Autodesk Fusion 360 part; units mm, degrees
(part 2 of 15)
  spline S3 degree 5 poles (-5.901, -3.7653) (-5.899, -3.7655) (-5.8948, -3.7657) (-5.8885, -3.7661) (-5.8802, -3.7667) (-5.8698, -3.7673) (-5.8594, -3.7679) (-5.849, -3.7685) (-5.8387, -3.769) (-5.8284, -3.7695) (-5.8181, -3.77) (-5.8079, -3.7705) (-5.7976, -3.7709) (-5.7874, -3.7713) (-5.7772, -3.7717) (-5.7671, -3.772) (-5.757, -3.7724) (-5.7468, -3.7727) (-5.7368, -3.7729) (-5.7267, -3.7732) (-5.7167, -3.7734) (-5.7067, -3.7736) (-5.6967, -3.7738) (-5.6868, -3.7739) (-5.6769, -3.774) (-5.667, -3.7741) (-5.6571, -3.7742) (-5.6473, -3.7742) (-5.6375, -3.7742) (-5.6277, -3.7742) (-5.6179, -3.7741) (-5.6082, -3.7741) (-5.5985, -3.774) (-5.5888, -3.7739) (-5.5792, -3.7737) (-5.5696, -3.7736) (-5.56, -3.7734) (-5.5504, -3.7732) (-5.5409, -3.7729) (-5.5314, -3.7727) (-5.5219, -3.7724) (-5.5125, -3.7721) (-5.5031, -3.7717) (-5.4937, -3.7714) (-5.4843, -3.771) (-5.475, -3.7706) (-5.4657, -3.7702) (-5.4565, -3.7697) (-5.4472, -3.7692) (-5.438, -3.7687) (-5.4289, -3.7682) (-5.4197, -3.7677) (-5.4106, -3.7671) (-5.4015, -3.7665) (-5.3925, -3.7659) (-5.3835, -3.7653) (-5.3745, -3.7646) (-5.3655, -3.764) (-5.3566, -3.7633) (-5.3477, -3.7625) (-5.3389, -3.7618) (-5.33, -3.761) (-5.3212, -3.7603) (-5.3125, -3.7594) (-5.3037, -3.7586) (-5.2951, -3.7578) (-5.2864, -3.7569) (-5.2778, -3.756) (-5.2692, -3.7551) (-5.2606, -3.7542) (-5.2521, -3.7532) (-5.2436, -3.7523) (-5.2351, -3.7513) (-5.2267, -3.7503) (-5.2183, -3.7493) (-5.2099, -3.7482) (-5.2016, -3.7472) (-5.1933, -3.7461) (-5.1851, -3.745) (-5.1768, -3.7439) (-5.1687, -3.7427) (-5.1605, -3.7416) (-5.1524, -3.7404) (-5.1443, -3.7392) (-5.1363, -3.738) (-5.1283, -3.7368) (-5.1203, -3.7355) (-5.1123, -3.7343) (-5.1044, -3.733) (-5.0966, -3.7317) (-5.0887, -3.7304) (-5.081, -3.7291) (-5.0732, -3.7277) (-5.0655, -3.7264) (-5.0578, -3.725) (-5.0502, -3.7236) (-5.0426, -3.7222) (-5.035, -3.7208) (-5.0275, -3.7194) (-5.02, -3.7179) (-5.0125, -3.7165) (-5.0051, -3.715) (-4.9977, -3.7135) (-4.9904, -3.712) (-4.9831, -3.7105) (-4.9758, -3.7089) (-4.9686, -3.7074) (-4.9614, -3.7058) (-4.9543, -3.7043) (-4.9472, -3.7027) (-4.9401, -3.7011) (-4.9331, -3.6995) (-4.9261, -3.6978) (-4.9191, -3.6962) (-4.9122, -3.6946) (-4.9054, -3.6929) (-4.8986, -3.6912) (-4.8918, -3.6896) (-4.885, -3.6879) (-4.8783, -3.6862) (-4.8717, -3.6845) (-4.8651, -3.6827) (-4.8585, -3.681) (-4.8519, -3.6793) (-4.8454, -3.6775) (-4.839, -3.6758) (-4.8326, -3.674) (-4.8262, -3.6722) (-4.8199, -3.6705) (-4.8136, -3.6687) (-4.8074, -3.6669) (-4.8012, -3.6651) (-4.795, -3.6632) (-4.7889, -3.6614) (-4.7829, -3.6596) (-4.7768, -3.6578) (-4.7709, -3.6559) (-4.7649, -3.6541) (-4.759, -3.6522) (-4.7532, -3.6504) (-4.7474, -3.6485) (-4.7416, -3.6466) (-4.7359, -3.6448) (-4.7303, -3.6429) (-4.7246, -3.641) (-4.7191, -3.6391) (-4.7135, -3.6373) (-4.708, -3.6354) (-4.7026, -3.6335) (-4.6972, -3.6316) (-4.6919, -3.6297) (-4.6866, -3.6278) (-4.6813, -3.6259) (-4.6761, -3.624) (-4.6709, -3.6221) (-4.6658, -3.6202) (-4.6608, -3.6183) (-4.6557, -3.6164) (-4.6508, -3.6145) (-4.6458, -3.6126) (-4.641, -3.6107) (-4.6361, -3.6088) (-4.6314, -3.6069) (-4.6266, -3.605) (-4.6219, -3.6031) (-4.6173, -3.6012) (-4.6127, -3.5993) (-4.6082, -3.5974) (-4.6037, -3.5955) (-4.5993, -3.5937) (-4.5949, -3.5918) (-4.5905, -3.5899) (-4.5863, -3.5881) (-4.582, -3.5862) (-4.5778, -3.5843) (-4.5737, -3.5825) (-4.5696, -3.5807) (-4.5656, -3.5788) (-4.5616, -3.577) (-4.5577, -3.5752) (-4.5538, -3.5734) (-4.5499, -3.5716) (-4.5462, -3.5698) (-4.5424, -3.568) (-4.5388, -3.5663) (-4.5351, -3.5645) (-4.5316, -3.5628) (-4.5281, -3.561) (-4.5246, -3.5593) (-4.5212, -3.5576) (-4.5178, -3.5559) (-4.5145, -3.5542) (-4.5113, -3.5525) (-4.5081, -3.5509) (-4.5049, -3.5492) (-4.5018, -3.5476) (-4.4988, -3.546) (-4.4958, -3.5444) (-4.4929, -3.5428) (-4.49, -3.5413) (-4.4872, -3.5397) (-4.4845, -3.5382) (-4.4818, -3.5367) (-4.4791, -3.5352) (-4.4765, -3.5338) (-4.474, -3.5323) (-4.4715, -3.5309) (-4.4691, -3.5295) (-4.4667, -3.5281) (-4.4644, -3.5267) (-4.4622, -3.5254) (-4.46, -3.5241) (-4.4579, -3.5228) (-4.4558, -3.5215) (-4.4538, -3.5203) (-4.4518, -3.5191) (-4.4499, -3.5179) (-4.4481, -3.5168) (-4.4463, -3.5156) (-4.4446, -3.5145) (-4.4429, -3.5135) (-4.4413, -3.5124) (-4.4398, -3.5114) (-4.4383, -3.5104) (-4.4369, -3.5095) (-4.4355, -3.5086) (-4.4342, -3.5077) (-4.433, -3.5069) (-4.4318, -3.5061) (-4.4307, -3.5053) (-4.4296, -3.5046) (-4.4286, -3.5039) (-4.4277, -3.5032) (-4.4268, -3.5026) (-4.426, -3.502) (-4.4253, -3.5015) (-4.4246, -3.501) (-4.424, -3.5005) (-4.4234, -3.5001) (-4.423, -3.4998) (-4.4225, -3.4994) (-4.4222, -3.4992) (-4.4221, -3.4991) (-4.422, -3.499) (-4.4219, -3.499) knots -1 -1 -1 -1 -1 -1 -0.99583333 -0.99166667 -0.9875 -0.98333333 -0.97916667 -0.975 -0.97083333 -0.96666667 -0.9625 -0.95833333 -0.95416667 -0.95 -0.94583333 -0.94166667 -0.9375 -0.93333333 -0.92916667 -0.925 -0.92083333 -0.91666667 -0.9125 -0.90833333 -0.90416667 -0.9 -0.89583333 -0.89166667 -0.8875 -0.88333333 -0.87916667 -0.875 -0.87083333 -0.86666667 -0.8625 -0.85833333 -0.85416667 -0.85 -0.84583333 -0.84166667 -0.8375 -0.83333333 -0.82916667 -0.825 -0.82083333 -0.81666667 -0.8125 -0.80833333 -0.80416667 -0.8 -0.79583333 -0.79166667 -0.7875 -0.78333333 -0.77916667 -0.775 -0.77083333 -0.76666667 -0.7625 -0.75833333 -0.75416667 -0.75 -0.74583333 -0.74166667 -0.7375 -0.73333333 -0.72916667 -0.725 -0.72083333 -0.71666667 -0.7125 -0.70833333 -0.70416667 -0.7 -0.69583333 -0.69166667 -0.6875 -0.68333333 -0.67916667 -0.675 -0.67083333 -0.66666667 -0.6625 -0.65833333 -0.65416667 -0.65 -0.64583333 -0.64166667 -0.6375 -0.63333333 -0.62916667 -0.625 -0.62083333 -0.61666667 -0.6125 -0.60833333 -0.60416667 -0.6 -0.59583333 -0.59166667 -0.5875 -0.58333333 -0.57916667 -0.575 -0.57083333 -0.56666667 -0.5625 -0.55833333 -0.55416667 -0.55 -0.54583333 -0.54166667 -0.5375 -0.53333333 -0.52916667 -0.525 -0.52083333 -0.51666667 -0.5125 -0.50833333 -0.50416667 -0.5 -0.49583333 -0.49166667 -0.4875 -0.48333333 -0.47916667 -0.475 -0.47083333 -0.46666667 -0.4625 -0.45833333 -0.45416667 -0.45 -0.44583333 -0.44166667 -0.4375 -0.43333333 -0.42916667 -0.425 -0.42083333 -0.41666667 -0.4125 -0.40833333 -0.40416667 -0.4 -0.39583333 -0.39166667 -0.3875 -0.38333333 -0.37916667 -0.375 -0.37083333 -0.36666667 -0.3625 -0.35833333 -0.35416667 -0.35 -0.34583333 -0.34166667 -0.3375 -0.33333333 -0.32916667 -0.325 -0.32083333 -0.31666667 -0.3125 -0.30833333 -0.30416667 -0.3 -0.29583333 -0.29166667 -0.2875 -0.28333333 -0.27916667 -0.275 -0.27083333 -0.26666667 -0.2625 -0.25833333 -0.25416667 -0.25 -0.24583333 -0.24166667 -0.2375 -0.23333333 -0.22916667 -0.225 -0.22083333 -0.21666667 -0.2125 -0.20833333 -0.20416667 -0.2 -0.19583333 -0.19166667 -0.1875 -0.18333333 -0.17916667 -0.175 -0.17083333 -0.16666667 -0.1625 -0.15833333 -0.15416667 -0.15 -0.14583333 -0.14166667 -0.1375 -0.13333333 -0.12916667 -0.125 -0.12083333 -0.11666667 -0.1125 -0.10833333 -0.10416667 -0.1 -0.09583333 -0.09166667 -0.0875 -0.08333333 -0.07916667 -0.075 -0.07083333 -0.06666667 -0.0625 -0.05833333 -0.05416667 -0.05 -0.04583333 -0.04166667 -0.0375 -0.03333333 -0.02916667 -0.025 -0.02083333 -0.01666667 -0.0125 -0.00833333 -0.00416667 0 0 0 0 0 0
  line L6 (-4.4219, -3.499) -> (-4.4214, -3.4986)
  line L7 (-4.4214, -3.4986) -> (-3.7249, -2.9475)
  arc A4 (-3.7249, -2.9475) -> (-2.9475, -3.7249) centre (0, 0) ccw
  line L8 (-2.9475, -3.7249) -> (-3.4986, -4.4214)
  line L9 (-3.4986, -4.4214) -> (-3.499, -4.4219)
  spline S4 degree 5 poles (-3.499, -4.4219) (-3.499, -4.422) (-3.4991, -4.4221) (-3.4992, -4.4222) (-3.4994, -4.4225) (-3.4998, -4.423) (-3.5001, -4.4234) (-3.5005, -4.424) (-3.501, -4.4246) (-3.5015, -4.4253) (-3.502, -4.426) (-3.5026, -4.4268) (-3.5032, -4.4277) (-3.5039, -4.4286) (-3.5046, -4.4296) (-3.5053, -4.4307) (-3.5061, -4.4318) (-3.5069, -4.433) (-3.5077, -4.4342) (-3.5086, -4.4355) (-3.5095, -4.4369) (-3.5104, -4.4383) (-3.5114, -4.4398) (-3.5124, -4.4413) (-3.5135, -4.4429) (-3.5145, -4.4446) (-3.5156, -4.4463) (-3.5168, -4.4481) (-3.5179, -4.4499) (-3.5191, -4.4518) (-3.5203, -4.4538) (-3.5215, -4.4558) (-3.5228, -4.4579) (-3.5241, -4.46) (-3.5254, -4.4622) (-3.5267, -4.4644) (-3.5281, -4.4667) (-3.5295, -4.4691) (-3.5309, -4.4715) (-3.5323, -4.474) (-3.5338, -4.4765) (-3.5352, -4.4791) (-3.5367, -4.4818) (-3.5382, -4.4845) (-3.5397, -4.4872) (-3.5413, -4.49) (-3.5428, -4.4929) (-3.5444, -4.4958) (-3.546, -4.4988) (-3.5476, -4.5018) (-3.5492, -4.5049) (-3.5509, -4.5081) (-3.5525, -4.5113) (-3.5542, -4.5145) (-3.5559, -4.5178) (-3.5576, -4.5212) (-3.5593, -4.5246) (-3.561, -4.5281) (-3.5628, -4.5316) (-3.5645, -4.5351) (-3.5663, -4.5388) (-3.568, -4.5424) (-3.5698, -4.5462) (-3.5716, -4.5499) (-3.5734, -4.5538) (-3.5752, -4.5577) (-3.577, -4.5616) (-3.5788, -4.5656) (-3.5807, -4.5696) (-3.5825, -4.5737) (-3.5843, -4.5778) (-3.5862, -4.582) (-3.5881, -4.5863) (-3.5899, -4.5905) (-3.5918, -4.5949) (-3.5937, -4.5993) (-3.5955, -4.6037) (-3.5974, -4.6082) (-3.5993, -4.6127) (-3.6012, -4.6173) (-3.6031, -4.6219) (-3.605, -4.6266) (-3.6069, -4.6314) (-3.6088, -4.6361) (-3.6107, -4.641) (-3.6126, -4.6458) (-3.6145, -4.6508) (-3.6164, -4.6557) (-3.6183, -4.6608) (-3.6202, -4.6658) (-3.6221, -4.6709) (-3.624, -4.6761) (-3.6259, -4.6813) (-3.6278, -4.6866) (-3.6297, -4.6919) (-3.6316, -4.6972) (-3.6335, -4.7026) (-3.6354, -4.708) (-3.6373, -4.7135) (-3.6391, -4.7191) (-3.641, -4.7246) (-3.6429, -4.7303) (-3.6448, -4.7359) (-3.6466, -4.7416) (-3.6485, -4.7474) (-3.6504, -4.7532) (-3.6522, -4.759) (-3.6541, -4.7649) (-3.6559, -4.7709) (-3.6578, -4.7768) (-3.6596, -4.7829) (-3.6614, -4.7889) (-3.6632, -4.795) (-3.6651, -4.8012) (-3.6669, -4.8074) (-3.6687, -4.8136) (-3.6705, -4.8199) (-3.6722, -4.8262) (-3.674, -4.8326) (-3.6758, -4.839) (-3.6775, -4.8454) (-3.6793, -4.8519) (-3.681, -4.8585) (-3.6827, -4.8651) (-3.6845, -4.8717) (-3.6862, -4.8783) (-3.6879, -4.885) (-3.6896, -4.8918) (-3.6912, -4.8986) (-3.6929, -4.9054) (-3.6946, -4.9122) (-3.6962, -4.9191) (-3.6978, -4.9261) (-3.6995, -4.9331) (-3.7011, -4.9401) (-3.7027, -4.9472) (-3.7043, -4.9543) (-3.7058, -4.9614) (-3.7074, -4.9686) (-3.7089, -4.9758) (-3.7105, -4.9831) (-3.712, -4.9904) (-3.7135, -4.9977) (-3.715, -5.0051) (-3.7165, -5.0125) (-3.7179, -5.02) (-3.7194, -5.0275) (-3.7208, -5.035) (-3.7222, -5.0426) (-3.7236, -5.0502) (-3.725, -5.0578) (-3.7264, -5.0655) (-3.7277, -5.0732) (-3.7291, -5.081) (-3.7304, -5.0887) (-3.7317, -5.0966) (-3.733, -5.1044) (-3.7343, -5.1123) (-3.7355, -5.1203) (-3.7368, -5.1283) (-3.738, -5.1363) (-3.7392, -5.1443) (-3.7404, -5.1524) (-3.7416, -5.1605) (-3.7427, -5.1687) (-3.7439, -5.1768) (-3.745, -5.1851) (-3.7461, -5.1933) (-3.7472, -5.2016) (-3.7482, -5.2099) (-3.7493, -5.2183) (-3.7503, -5.2267) (-3.7513, -5.2351) (-3.7523, -5.2436) (-3.7532, -5.2521) (-3.7542, -5.2606) (-3.7551, -5.2692) (-3.756, -5.2778) (-3.7569, -5.2864) (-3.7578, -5.2951) (-3.7586, -5.3037) (-3.7594, -5.3125) (-3.7603, -5.3212) (-3.761, -5.33) (-3.7618, -5.3389) (-3.7625, -5.3477) (-3.7633, -5.3566) (-3.764, -5.3655) (-3.7646, -5.3745) (-3.7653, -5.3835) (-3.7659, -5.3925) (-3.7665, -5.4015) (-3.7671, -5.4106) (-3.7677, -5.4197) (-3.7682, -5.4289) (-3.7687, -5.438) (-3.7692, -5.4472) (-3.7697, -5.4565) (-3.7702, -5.4657) (-3.7706, -5.475) (-3.771, -5.4843) (-3.7714, -5.4937) (-3.7717, -5.5031) (-3.7721, -5.5125) (-3.7724, -5.5219) (-3.7727, -5.5314) (-3.7729, -5.5409) (-3.7732, -5.5504) (-3.7734, -5.56) (-3.7736, -5.5696) (-3.7737, -5.5792) (-3.7739, -5.5888) (-3.774, -5.5985) (-3.7741, -5.6082) (-3.7741, -5.6179) (-3.7742, -5.6277) (-3.7742, -5.6375) (-3.7742, -5.6473) (-3.7742, -5.6571) (-3.7741, -5.667) (-3.774, -5.6769) (-3.7739, -5.6868) (-3.7738, -5.6967) (-3.7736, -5.7067) (-3.7734, -5.7167) (-3.7732, -5.7267) (-3.7729, -5.7368) (-3.7727, -5.7468) (-3.7724, -5.757) (-3.772, -5.7671) (-3.7717, -5.7772) (-3.7713, -5.7874) (-3.7709, -5.7976) (-3.7705, -5.8079) (-3.77, -5.8181) (-3.7695, -5.8284) (-3.769, -5.8387) (-3.7685, -5.849) (-3.7679, -5.8594) (-3.7673, -5.8698) (-3.7667, -5.8802) (-3.7661, -5.8885) (-3.7657, -5.8948) (-3.7655, -5.899) (-3.7653, -5.901) knots 0 0 0 0 0 0 0.00416667 0.00833333 0.0125 0.01666667 0.02083333 0.025 0.02916667 0.03333333 0.0375 0.04166667 0.04583333 0.05 0.05416667 0.05833333 0.0625 0.06666667 0.07083333 0.075 0.07916667 0.08333333 0.0875 0.09166667 0.09583333 0.1 0.10416667 0.10833333 0.1125 0.11666667 0.12083333 0.125 0.12916667 0.13333333 0.1375 0.14166667 0.14583333 0.15 0.15416667 0.15833333 0.1625 0.16666667 0.17083333 0.175 0.17916667 0.18333333 0.1875 0.19166667 0.19583333 0.2 0.20416667 0.20833333 0.2125 0.21666667 0.22083333 0.225 0.22916667 0.23333333 0.2375 0.24166667 0.24583333 0.25 0.25416667 0.25833333 0.2625 0.26666667 0.27083333 0.275 0.27916667 0.28333333 0.2875 0.29166667 0.29583333 0.3 0.30416667 0.30833333 0.3125 0.31666667 0.32083333 0.325 0.32916667 0.33333333 0.3375 0.34166667 0.34583333 0.35 0.35416667 0.35833333 0.3625 0.36666667 0.37083333 0.375 0.37916667 0.38333333 0.3875 0.39166667 0.39583333 0.4 0.40416667 0.40833333 0.4125 0.41666667 0.42083333 0.425 0.42916667 0.43333333 0.4375 0.44166667 0.44583333 0.45 0.45416667 0.45833333 0.4625 0.46666667 0.47083333 0.475 0.47916667 0.48333333 0.4875 0.49166667 0.49583333 0.5 0.50416667 0.50833333 0.5125 0.51666667 0.52083333 0.525 0.52916667 0.53333333 0.5375 0.54166667 0.54583333 0.55 0.55416667 0.55833333 0.5625 0.56666667 0.57083333 0.575 0.57916667 0.58333333 0.5875 0.59166667 0.59583333 0.6 0.60416667 0.60833333 0.6125 0.61666667 0.62083333 0.625 0.62916667 0.63333333 0.6375 0.64166667 0.64583333 0.65 0.65416667 0.65833333 0.6625 0.66666667 0.67083333 0.675 0.67916667 0.68333333 0.6875 0.69166667 0.69583333 0.7 0.70416667 0.70833333 0.7125 0.71666667 0.72083333 0.725 0.72916667 0.73333333 0.7375 0.74166667 0.74583333 0.75 0.75416667 0.75833333 0.7625 0.76666667 0.77083333 0.775 0.77916667 0.78333333 0.7875 0.79166667 0.79583333 0.8 0.80416667 0.80833333 0.8125 0.81666667 0.82083333 0.825 0.82916667 0.83333333 0.8375 0.84166667 0.84583333 0.85 0.85416667 0.85833333 0.8625 0.86666667 0.87083333 0.875 0.87916667 0.88333333 0.8875 0.89166667 0.89583333 0.9 0.90416667 0.90833333 0.9125 0.91666667 0.92083333 0.925 0.92916667 0.93333333 0.9375 0.94166667 0.94583333 0.95 0.95416667 0.95833333 0.9625 0.96666667 0.97083333 0.975 0.97916667 0.98333333 0.9875 0.99166667 0.99583333 1 1 1 1 1 1
  arc A5 (-3.7653, -5.901) -> (-3.2278, -6.2114) centre (0, 0) ccw
  spline S5 degree 5 poles (-3.2278, -6.2114) (-3.2259, -6.2105) (-3.2221, -6.2086) (-3.2165, -6.2058) (-3.209, -6.2021) (-3.1997, -6.1975) (-3.1904, -6.1928) (-3.1812, -6.1881) (-3.172, -6.1834) (-3.1628, -6.1787) (-3.1536, -6.174) (-3.1445, -6.1692) (-3.1354, -6.1645) (-3.1264, -6.1598) (-3.1174, -6.155) (-3.1084, -6.1502) (-3.0995, -6.1454) (-3.0906, -6.1406) (-3.0817, -6.1358) (-3.0729, -6.131) (-3.0641, -6.1262) (-3.0554, -6.1214) (-3.0466, -6.1165) (-3.038, -6.1117) (-3.0293, -6.1068) (-3.0207, -6.1019) (-3.0121, -6.0971) (-3.0036, -6.0922) (-2.9951, -6.0873) (-2.9866, -6.0824) (-2.9782, -6.0775) (-2.9698, -6.0726) (-2.9614, -6.0676) (-2.9531, -6.0627) (-2.9448, -6.0577) (-2.9366, -6.0528) (-2.9284, -6.0478) (-2.9202, -6.0429) (-2.9121, -6.0379) (-2.904, -6.0329) (-2.8959, -6.0279) (-2.8879, -6.023) (-2.8799, -6.018) (-2.872, -6.013) (-2.8641, -6.008) (-2.8562, -6.0029) (-2.8484, -5.9979) (-2.8406, -5.9929) (-2.8328, -5.9879) (-2.8251, -5.9828) (-2.8174, -5.9778) (-2.8098, -5.9728) (-2.8022, -5.9677) (-2.7946, -5.9627) (-2.7871, -5.9576) (-2.7796, -5.9526) (-2.7721, -5.9475) (-2.7647, -5.9424) (-2.7573, -5.9374) (-2.75, -5.9323) (-2.7427, -5.9272) (-2.7354, -5.9222) (-2.7282, -5.9171) (-2.721, -5.912) (-2.7139, -5.9069) (-2.7068, -5.9019) (-2.6997, -5.8968) (-2.6927, -5.8917) (-2.6857, -5.8866) (-2.6787, -5.8815) (-2.6718, -5.8764) (-2.6649, -5.8714) (-2.6581, -5.8663) (-2.6513, -5.8612) (-2.6445, -5.8561) (-2.6378, -5.851) (-2.6311, -5.8459) (-2.6245, -5.8409) (-2.6179, -5.8358) (-2.6113, -5.8307) (-2.6048, -5.8256) (-2.5983, -5.8205) (-2.5919, -5.8155) (-2.5855, -5.8104) (-2.5791, -5.8053) (-2.5728, -5.8003) (-2.5665, -5.7952) (-2.5603, -5.7902) (-2.5541, -5.7851) (-2.5479, -5.78) (-2.5418, -5.775) (-2.5357, -5.77) (-2.5297, -5.7649) (-2.5236, -5.7599) (-2.5177, -5.7549) (-2.5118, -5.7498) (-2.5059, -5.7448) (-2.5, -5.7398) (-2.4942, -5.7348) (-2.4885, -5.7298) (-2.4827, -5.7248) (-2.4771, -5.7198) (-2.4714, -5.7148) (-2.4658, -5.7099) (-2.4602, -5.7049) (-2.4547, -5.6999) (-2.4492, -5.695) (-2.4438, -5.69) (-2.4384, -5.6851) (-2.433, -5.6802) (-2.4277, -5.6753) (-2.4224, -5.6704) (-2.4172, -5.6655) (-2.412, -5.6606) (-2.4068, -5.6557) (-2.4017, -5.6508) (-2.3967, -5.646) (-2.3916, -5.6411) (-2.3866, -5.6363) (-2.3817, -5.6315) (-2.3768, -5.6267) (-2.3719, -5.6219) (-2.3671, -5.6171) (-2.3623, -5.6123) (-2.3575, -5.6076) (-2.3528, -5.6028) (-2.3481, -5.5981) (-2.3435, -5.5934) (-2.3389, -5.5887) (-2.3344, -5.584) (-2.3299, -5.5793) (-2.3254, -5.5746) (-2.321, -5.57) (-2.3166, -5.5653) (-2.3123, -5.5607) (-2.308, -5.5561) (-2.3037, -5.5516) (-2.2995, -5.547) (-2.2953, -5.5424) (-2.2912, -5.5379) (-2.2871, -5.5334) (-2.283, -5.5289) (-2.279, -5.5244) (-2.2751, -5.52) (-2.2711, -5.5155) (-2.2673, -5.5111) (-2.2634, -5.5067) (-2.2596, -5.5023) (-2.2558, -5.498) (-2.2521, -5.4936) (-2.2484, -5.4893) (-2.2448, -5.485) (-2.2412, -5.4808) (-2.2376, -5.4765) (-2.2341, -5.4723) (-2.2306, -5.4681) (-2.2272, -5.4639) (-2.2238, -5.4597) (-2.2204, -5.4556) (-2.2171, -5.4515) (-2.2139, -5.4474) (-2.2106, -5.4434) (-2.2074, -5.4393) (-2.2043, -5.4353) (-2.2012, -5.4313) (-2.1981, -5.4274) (-2.1951, -5.4234) (-2.1921, -5.4195) (-2.1892, -5.4157) (-2.1863, -5.4118) (-2.1834, -5.408) (-2.1806, -5.4042) (-2.1778, -5.4005) (-2.175, -5.3967) (-2.1723, -5.393) (-2.1697, -5.3894) (-2.1671, -5.3858) (-2.1645, -5.3821) (-2.1619, -5.3786) (-2.1594, -5.375) (-2.157, -5.3715) (-2.1546, -5.3681) (-2.1522, -5.3646) (-2.1498, -5.3612) (-2.1475, -5.3579) (-2.1453, -5.3545) (-2.1431, -5.3512) (-2.1409, -5.348) (-2.1388, -5.3447) (-2.1367, -5.3416) (-2.1346, -5.3384) (-2.1326, -5.3353) (-2.1306, -5.3322) (-2.1287, -5.3292) (-2.1268, -5.3262) (-2.1249, -5.3233) (-2.1231, -5.3203) (-2.1213, -5.3175) (-2.1196, -5.3146) (-2.1179, -5.3119) (-2.1162, -5.3091) (-2.1146, -5.3064) (-2.113, -5.3038) (-2.1114, -5.3012) (-2.1099, -5.2986) (-2.1084, -5.2961) (-2.107, -5.2936) (-2.1056, -5.2912) (-2.1043, -5.2888) (-2.1029, -5.2865) (-2.1017, -5.2842) (-2.1004, -5.2819) (-2.0992, -5.2798) (-2.0981, -5.2776) (-2.0969, -5.2756) (-2.0958, -5.2735) (-2.0948, -5.2716) (-2.0938, -5.2696) (-2.0928, -5.2678) (-2.0918, -5.266) (-2.0909, -5.2642) (-2.0901, -5.2625) (-2.0892, -5.2609) (-2.0884, -5.2593) (-2.0877, -5.2577) (-2.087, -5.2563) (-2.0863, -5.2549) (-2.0856, -5.2535) (-2.085, -5.2522) (-2.0844, -5.251) (-2.0839, -5.2498) (-2.0834, -5.2487) (-2.0829, -5.2477) (-2.0824, -5.2467) (-2.082, -5.2458) (-2.0817, -5.245) (-2.0813, -5.2442) (-2.081, -5.2435) (-2.0807, -5.2429) (-2.0805, -5.2424) (-2.0803, -5.2419) (-2.0802, -5.2415) (-2.0801, -5.2413) (-2.08, -5.2412) (-2.08, -5.2411) knots -1 -1 -1 -1 -1 -1 -0.99583333 -0.99166667 -0.9875 -0.98333333 -0.97916667 -0.975 -0.97083333 -0.96666667 -0.9625 -0.95833333 -0.95416667 -0.95 -0.94583333 -0.94166667 -0.9375 -0.93333333 -0.92916667 -0.925 -0.92083333 -0.91666667 -0.9125 -0.90833333 -0.90416667 -0.9 -0.89583333 -0.89166667 -0.8875 -0.88333333 -0.87916667 -0.875 -0.87083333 -0.86666667 -0.8625 -0.85833333 -0.85416667 -0.85 -0.84583333 -0.84166667 -0.8375 -0.83333333 -0.82916667 -0.825 -0.82083333 -0.81666667 -0.8125 -0.80833333 -0.80416667 -0.8 -0.79583333 -0.79166667 -0.7875 -0.78333333 -0.77916667 -0.775 -0.77083333 -0.76666667 -0.7625 -0.75833333 -0.75416667 -0.75 -0.74583333 -0.74166667 -0.7375 -0.73333333 -0.72916667 -0.725 -0.72083333 -0.71666667 -0.7125 -0.70833333 -0.70416667 -0.7 -0.69583333 -0.69166667 -0.6875 -0.68333333 -0.67916667 -0.675 -0.67083333 -0.66666667 -0.6625 -0.65833333 -0.65416667 -0.65 -0.64583333 -0.64166667 -0.6375 -0.63333333 -0.62916667 -0.625 -0.62083333 -0.61666667 -0.6125 -0.60833333 -0.60416667 -0.6 -0.59583333 -0.59166667 -0.5875 -0.58333333 -0.57916667 -0.575 -0.57083333 -0.56666667 -0.5625 -0.55833333 -0.55416667 -0.55 -0.54583333 -0.54166667 -0.5375 -0.53333333 -0.52916667 -0.525 -0.52083333 -0.51666667 -0.5125 -0.50833333 -0.50416667 -0.5 -0.49583333 -0.49166667 -0.4875 -0.48333333 -0.47916667 -0.475 -0.47083333 -0.46666667 -0.4625 -0.45833333 -0.45416667 -0.45 -0.44583333 -0.44166667 -0.4375 -0.43333333 -0.42916667 -0.425 -0.42083333 -0.41666667 -0.4125 -0.40833333 -0.40416667 -0.4 -0.39583333 -0.39166667 -0.3875 -0.38333333 -0.37916667 -0.375 -0.37083333 -0.36666667 -0.3625 -0.35833333 -0.35416667 -0.35 -0.34583333 -0.34166667 -0.3375 -0.33333333 -0.32916667 -0.325 -0.32083333 -0.31666667 -0.3125 -0.30833333 -0.30416667 -0.3 -0.29583333 -0.29166667 -0.2875 -0.28333333 -0.27916667 -0.275 -0.27083333 -0.26666667 -0.2625 -0.25833333 -0.25416667 -0.25 -0.24583333 -0.24166667 -0.2375 -0.23333333 -0.22916667 -0.225 -0.22083333 -0.21666667 -0.2125 -0.20833333 -0.20416667 -0.2 -0.19583333 -0.19166667 -0.1875 -0.18333333 -0.17916667 -0.175 -0.17083333 -0.16666667 -0.1625 -0.15833333 -0.15416667 -0.15 -0.14583333 -0.14166667 -0.1375 -0.13333333 -0.12916667 -0.125 -0.12083333 -0.11666667 -0.1125 -0.10833333 -0.10416667 -0.1 -0.09583333 -0.09166667 -0.0875 -0.08333333 -0.07916667 -0.075 -0.07083333 -0.06666667 -0.0625 -0.05833333 -0.05416667 -0.05 -0.04583333 -0.04166667 -0.0375 -0.03333333 -0.02916667 -0.025 -0.02083333 -0.01666667 -0.0125 -0.00833333 -0.00416667 0 0 0 0 0 0
  line L10 (-2.08, -5.2411) -> (-2.0798, -5.2406)
  line L11 (-2.0798, -5.2406) -> (-1.7521, -4.415)
  arc A6 (-1.7521, -4.415) -> (-0.6901, -4.6996) centre (0, 0) ccw
  line L12 (-0.6901, -4.6996) -> (-0.8192, -5.5783)
  line L13 (-0.8192, -5.5783) -> (-0.8192, -5.579)
  spline S6 degree 5 poles (-0.8192, -5.579) (-0.8193, -5.579) (-0.8193, -5.5792) (-0.8193, -5.5794) (-0.8193, -5.5797) (-0.8194, -5.5803) (-0.8195, -5.5809) (-0.8196, -5.5815) (-0.8196, -5.5823) (-0.8197, -5.5831) (-0.8198, -5.584) (-0.8199, -5.585) (-0.82, -5.5861) (-0.8201, -5.5872) (-0.8202, -5.5884) (-0.8203, -5.5897) (-0.8204, -5.5911) (-0.8206, -5.5925) (-0.8207, -5.594) (-0.8208, -5.5955) (-0.8209, -5.5972) (-0.821, -5.5989) (-0.8211, -5.6007) (-0.8212, -5.6025) (-0.8213, -5.6044) (-0.8214, -5.6064) (-0.8215, -5.6084) (-0.8216, -5.6105) (-0.8216, -5.6127) (-0.8217, -5.6149) (-0.8218, -5.6172) (-0.8218, -5.6196) (-0.8219, -5.622) (-0.822, -5.6245) (-0.822, -5.6271) (-0.822, -5.6297) (-0.822, -5.6324) (-0.8221, -5.6351) (-0.8221, -5.6379) (-0.8221, -5.6408) (-0.8221, -5.6437) (-0.822, -5.6466) (-0.822, -5.6497) (-0.8219, -5.6528) (-0.8219, -5.6559) (-0.8218, -5.6591) (-0.8217, -5.6624) (-0.8216, -5.6657) (-0.8215, -5.6691) (-0.8214, -5.6725) (-0.8213, -5.676) (-0.8211, -5.6796) (-0.821, -5.6831) (-0.8208, -5.6868) (-0.8206, -5.6905) (-0.8204, -5.6943) (-0.8202, -5.6981) (-0.8199, -5.7019) (-0.8197, -5.7058) (-0.8194, -5.7098) (-0.8191, -5.7138) (-0.8188, -5.7179) (-0.8185, -5.722) (-0.8181, -5.7262) (-0.8178, -5.7304) (-0.8174, -5.7346) (-0.817, -5.739) (-0.8166, -5.7433) (-0.8161, -5.7477) (-0.8157, -5.7522) (-0.8152, -5.7567) (-0.8147, -5.7612) (-0.8142, -5.7658) (-0.8137, -5.7705) (-0.8131, -5.7752) (-0.8126, -5.7799) (-0.812, -5.7847) (-0.8114, -5.7895) (-0.8107, -5.7944) (-0.8101, -5.7993) (-0.8094, -5.8043) (-0.8087, -5.8093) (-0.808, -5.8143) (-0.8072, -5.8194) (-0.8064, -5.8245) (-0.8057, -5.8297) (-0.8048, -5.8349) (-0.804, -5.8402) (-0.8031, -5.8455) (-0.8023, -5.8508) (-0.8013, -5.8562) (-0.8004, -5.8616) (-0.7995, -5.8671) (-0.7985, -5.8726) (-0.7975, -5.8781) (-0.7964, -5.8837) (-0.7954, -5.8893) (-0.7943, -5.895) (-0.7932, -5.9007) (-0.7921, -5.9064) (-0.7909, -5.9122) (-0.7897, -5.918) (-0.7885, -5.9238) (-0.7873, -5.9297) (-0.786, -5.9356) (-0.7847, -5.9416) (-0.7834, -5.9476) (-0.7821, -5.9536) (-0.7807, -5.9596) (-0.7793, -5.9657) (-0.7779, -5.9719) (-0.7764, -5.978) (-0.7749, -5.9842) (-0.7734, -5.9905) (-0.7719, -5.9967) (-0.7703, -6.003) (-0.7688, -6.0094) (-0.7671, -6.0157) (-0.7655, -6.0221) (-0.7638, -6.0286) (-0.7621, -6.035) (-0.7604, -6.0415) (-0.7586, -6.0481) (-0.7568, -6.0546) (-0.755, -6.0612) (-0.7532, -6.0678) (-0.7513, -6.0745) (-0.7494, -6.0812) (-0.7474, -6.0879) (-0.7455, -6.0946) (-0.7435, -6.1014) (-0.7414, -6.1082) (-0.7394, -6.115) (-0.7373, -6.1219) (-0.7352, -6.1288) (-0.733, -6.1357) (-0.7308, -6.1427) (-0.7286, -6.1496) (-0.7264, -6.1566) (-0.7241, -6.1637) (-0.7218, -6.1707) (-0.7195, -6.1778) (-0.7171, -6.1849) (-0.7147, -6.192) (-0.7123, -6.1992) (-0.7098, -6.2064) (-0.7073, -6.2136) (-0.7048, -6.2208) (-0.7023, -6.2281) (-0.6997, -6.2354) (-0.6971, -6.2427) (-0.6944, -6.25) (-0.6917, -6.2574) (-0.689, -6.2648) (-0.6863, -6.2722) (-0.6835, -6.2796) (-0.6807, -6.2871) (-0.6778, -6.2946) (-0.6749, -6.3021) (-0.672, -6.3096) (-0.6691, -6.3171) (-0.6661, -6.3247) (-0.6631, -6.3323) (-0.66, -6.3399) (-0.657, -6.3475) (-0.6539, -6.3552) (-0.6507, -6.3629) (-0.6475, -6.3706) (-0.6443, -6.3783) (-0.6411, -6.386) (-0.6378, -6.3938) (-0.6345, -6.4016) (-0.6312, -6.4094) (-0.6278, -6.4172) (-0.6244, -6.4251) (-0.6209, -6.4329) (-0.6174, -6.4408) (-0.6139, -6.4487) (-0.6104, -6.4566) (-0.6068, -6.4645) (-0.6032, -6.4725) (-0.5995, -6.4805) (-0.5959, -6.4885) (-0.5921, -6.4965) (-0.5884, -6.5045) (-0.5846, -6.5125) (-0.5808, -6.5206) (-0.5769, -6.5287) (-0.573, -6.5368) (-0.5691, -6.5449) (-0.5651, -6.553) (-0.5611, -6.5611) (-0.5571, -6.5693) (-0.553, -6.5775) (-0.5489, -6.5856) (-0.5448, -6.5938) (-0.5406, -6.6021) (-0.5364, -6.6103) (-0.5322, -6.6185) (-0.5279, -6.6268) (-0.5236, -6.6351) (-0.5193, -6.6434) (-0.5149, -6.6517) (-0.5105, -6.66) (-0.506, -6.6683) (-0.5015, -6.6767) (-0.497, -6.685) (-0.4924, -6.6934) (-0.4879, -6.7018) (-0.4832, -6.7102) (-0.4786, -6.7186) (-0.4739, -6.727) (-0.4691, -6.7354) (-0.4644, -6.7439) (-0.4595, -6.7523) (-0.4547, -6.7608) (-0.4498, -6.7693) (-0.4449, -6.7778) (-0.44, -6.7863) (-0.435, -6.7948) (-0.43, -6.8033) (-0.4249, -6.8118) (-0.4198, -6.8204) (-0.4147, -6.8289) (-0.4095, -6.8375) (-0.4043, -6.8461) (-0.3991, -6.8547) (-0.3938, -6.8632) (-0.3885, -6.8718) (-0.3831, -6.8805) (-0.3778, -6.8891) (-0.3723, -6.8977) (-0.3669, -6.9063) (-0.3614, -6.915) (-0.3559, -6.9236) (-0.3503, -6.9323) (-0.3447, -6.941) (-0.3391, -6.9496) (-0.3334, -6.9583) (-0.3277, -6.967) (-0.322, -6.9757) (-0.3173, -6.9827) (-0.3138, -6.9879) (-0.3115, -6.9914) (-0.3103, -6.9931) knots 0 0 0 0 0 0 0.00416667 0.00833333 0.0125 0.01666667 0.02083333 0.025 0.02916667 0.03333333 0.0375 0.04166667 0.04583333 0.05 0.05416667 0.05833333 0.0625 0.06666667 0.07083333 0.075 0.07916667 0.08333333 0.0875 0.09166667 0.09583333 0.1 0.10416667 0.10833333 0.1125 0.11666667 0.12083333 0.125 0.12916667 0.13333333 0.1375 0.14166667 0.14583333 0.15 0.15416667 0.15833333 0.1625 0.16666667 0.17083333 0.175 0.17916667 0.18333333 0.1875 0.19166667 0.19583333 0.2 0.20416667 0.20833333 0.2125 0.21666667 0.22083333 0.225 0.22916667 0.23333333 0.2375 0.24166667 0.24583333 0.25 0.25416667 0.25833333 0.2625 0.26666667 0.27083333 0.275 0.27916667 0.28333333 0.2875 0.29166667 0.29583333 0.3 0.30416667 0.30833333 0.3125 0.31666667 0.32083333 0.325 0.32916667 0.33333333 0.3375 0.34166667 0.34583333 0.35 0.35416667 0.35833333 0.3625 0.36666667 0.37083333 0.375 0.37916667 0.38333333 0.3875 0.39166667 0.39583333 0.4 0.40416667 0.40833333 0.4125 0.41666667 0.42083333 0.425 0.42916667 0.43333333 0.4375 0.44166667 0.44583333 0.45 0.45416667 0.45833333 0.4625 0.46666667 0.47083333 0.475 0.47916667 0.48333333 0.4875 0.49166667 0.49583333 0.5 0.50416667 0.50833333 0.5125 0.51666667 0.52083333 0.525 0.52916667 0.53333333 0.5375 0.54166667 0.54583333 0.55 0.55416667 0.55833333 0.5625 0.56666667 0.57083333 0.575 0.57916667 0.58333333 0.5875 0.59166667 0.59583333 0.6 0.60416667 0.60833333 0.6125 0.61666667 0.62083333 0.625 0.62916667 0.63333333 0.6375 0.64166667 0.64583333 0.65 0.65416667 0.65833333 0.6625 0.66666667 0.67083333 0.675 0.67916667 0.68333333 0.6875 0.69166667 0.69583333 0.7 0.70416667 0.70833333 0.7125 0.71666667 0.72083333 0.725 0.72916667 0.73333333 0.7375 0.74166667 0.74583333 0.75 0.75416667 0.75833333 0.7625 0.76666667 0.77083333 0.775 0.77916667 0.78333333 0.7875 0.79166667 0.79583333 0.8 0.80416667 0.80833333 0.8125 0.81666667 0.82083333 0.825 0.82916667 0.83333333 0.8375 0.84166667 0.84583333 0.85 0.85416667 0.85833333 0.8625 0.86666667 0.87083333 0.875 0.87916667 0.88333333 0.8875 0.89166667 0.89583333 0.9 0.90416667 0.90833333 0.9125 0.91666667 0.92083333 0.925 0.92916667 0.93333333 0.9375 0.94166667 0.94583333 0.95 0.95416667 0.95833333 0.9625 0.96666667 0.97083333 0.975 0.97916667 0.98333333 0.9875 0.99166667 0.99583333 1 1 1 1 1 1
  arc A7 (-0.3103, -6.9931) -> (0.3103, -6.9931) centre (0, 0) ccw
  spline S7 degree 5 poles (0.3103, -6.9931) (0.3115, -6.9914) (0.3138, -6.9879) (0.3173, -6.9827) (0.322, -6.9757) (0.3277, -6.967) (0.3334, -6.9583) (0.3391, -6.9496) (0.3447, -6.941) (0.3503, -6.9323) (0.3559, -6.9236) (0.3614, -6.915) (0.3669, -6.9063) (0.3723, -6.8977) (0.3778, -6.8891) (0.3831, -6.8805) (0.3885, -6.8718) (0.3938, -6.8632) (0.3991, -6.8547) (0.4043, -6.8461) (0.4095, -6.8375) (0.4147, -6.8289) (0.4198, -6.8204) (0.4249, -6.8118) (0.43, -6.8033) (0.435, -6.7948) (0.44, -6.7863) (0.4449, -6.7778) (0.4498, -6.7693) (0.4547, -6.7608) (0.4595, -6.7523) (0.4644, -6.7439) (0.4691, -6.7354) (0.4739, -6.727) (0.4786, -6.7186) (0.4832, -6.7102) (0.4879, -6.7018) (0.4924, -6.6934) (0.497, -6.685) (0.5015, -6.6767) (0.506, -6.6683) (0.5105, -6.66) (0.5149, -6.6517) (0.5193, -6.6434) (0.5236, -6.6351) (0.5279, -6.6268) (0.5322, -6.6185) (0.5364, -6.6103) (0.5406, -6.6021) (0.5448, -6.5938) (0.5489, -6.5856) (0.553, -6.5775) (0.5571, -6.5693) (0.5611, -6.5611) (0.5651, -6.553) (0.5691, -6.5449) (0.573, -6.5368) (0.5769, -6.5287) (0.5808, -6.5206) (0.5846, -6.5125) (0.5884, -6.5045) (0.5921, -6.4965) (0.5959, -6.4885) (0.5995, -6.4805) (0.6032, -6.4725) (0.6068, -6.4645) (0.6104, -6.4566) (0.6139, -6.4487) (0.6174, -6.4408) (0.6209, -6.4329) (0.6244, -6.4251) (0.6278, -6.4172) (0.6312, -6.4094) (0.6345, -6.4016) (0.6378, -6.3938) (0.6411, -6.386) (0.6443, -6.3783) (0.6475, -6.3706) (0.6507, -6.3629) (0.6539, -6.3552) (0.657, -6.3475) (0.66, -6.3399) (0.6631, -6.3323) (0.6661, -6.3247) (0.6691, -6.3171) (0.672, -6.3096) (0.6749, -6.3021) (0.6778, -6.2946) (0.6807, -6.2871) (0.6835, -6.2796) (0.6863, -6.2722) (0.689, -6.2648) (0.6917, -6.2574) (0.6944, -6.25) (0.6971, -6.2427) (0.6997, -6.2354) (0.7023, -6.2281) (0.7048, -6.2208) (0.7073, -6.2136) (0.7098, -6.2064) (0.7123, -6.1992) (0.7147, -6.192) (0.7171, -6.1849) (0.7195, -6.1778) (0.7218, -6.1707) (0.7241, -6.1637) (0.7264, -6.1566) (0.7286, -6.1496) (0.7308, -6.1427) (0.733, -6.1357) (0.7352, -6.1288) (0.7373, -6.1219) (0.7394, -6.115) (0.7414, -6.1082) (0.7435, -6.1014) (0.7455, -6.0946) (0.7474, -6.0879) (0.7494, -6.0812) (0.7513, -6.0745) (0.7532, -6.0678) (0.755, -6.0612) (0.7568, -6.0546) (0.7586, -6.0481) (0.7604, -6.0415) (0.7621, -6.035) (0.7638, -6.0286) (0.7655, -6.0221) (0.7671, -6.0157) (0.7688, -6.0094) (0.7703, -6.003) (0.7719, -5.9967) (0.7734, -5.9905) (0.7749, -5.9842) (0.7764, -5.978) (0.7779, -5.9719) (0.7793, -5.9657) (0.7807, -5.9596) (0.7821, -5.9536) (0.7834, -5.9476) (0.7847, -5.9416) (0.786, -5.9356) (0.7873, -5.9297) (0.7885, -5.9238) (0.7897, -5.918) (0.7909, -5.9122) (0.7921, -5.9064) (0.7932, -5.9007) (0.7943, -5.895) (0.7954, -5.8893) (0.7964, -5.8837) (0.7975, -5.8781) (0.7985, -5.8726) (0.7995, -5.8671) (0.8004, -5.8616) (0.8013, -5.8562) (0.8023, -5.8508) (0.8031, -5.8455) (0.804, -5.8402) (0.8048, -5.8349) (0.8057, -5.8297) (0.8064, -5.8245) (0.8072, -5.8194) (0.808, -5.8143) (0.8087, -5.8093) (0.8094, -5.8043) (0.8101, -5.7993) (0.8107, -5.7944) (0.8114, -5.7895) (0.812, -5.7847) (0.8126, -5.7799) (0.8131, -5.7752) (0.8137, -5.7705) (0.8142, -5.7658) (0.8147, -5.7612) (0.8152, -5.7567) (0.8157, -5.7522) (0.8161, -5.7477) (0.8166, -5.7433) (0.817, -5.739) (0.8174, -5.7346) (0.8178, -5.7304) (0.8181, -5.7262) (0.8185, -5.722) (0.8188, -5.7179) (0.8191, -5.7138) (0.8194, -5.7098) (0.8197, -5.7058) (0.8199, -5.7019) (0.8202, -5.6981) (0.8204, -5.6943) (0.8206, -5.6905) (0.8208, -5.6868) (0.821, -5.6831) (0.8211, -5.6796) (0.8213, -5.676) (0.8214, -5.6725) (0.8215, -5.6691) (0.8216, -5.6657) (0.8217, -5.6624) (0.8218, -5.6591) (0.8219, -5.6559) (0.8219, -5.6528) (0.822, -5.6497) (0.822, -5.6466) (0.8221, -5.6437) (0.8221, -5.6408) (0.8221, -5.6379) (0.8221, -5.6351) (0.822, -5.6324) (0.822, -5.6297) (0.822, -5.6271) (0.822, -5.6245) (0.8219, -5.622) (0.8218, -5.6196) (0.8218, -5.6172) (0.8217, -5.6149) (0.8216, -5.6127) (0.8216, -5.6105) (0.8215, -5.6084) (0.8214, -5.6064) (0.8213, -5.6044) (0.8212, -5.6025) (0.8211, -5.6007) (0.821, -5.5989) (0.8209, -5.5972) (0.8208, -5.5955) (0.8207, -5.594) (0.8206, -5.5925) (0.8204, -5.5911) (0.8203, -5.5897) (0.8202, -5.5884) (0.8201, -5.5872) (0.82, -5.5861) (0.8199, -5.585) (0.8198, -5.584) (0.8197, -5.5831) (0.8196, -5.5823) (0.8196, -5.5815) (0.8195, -5.5809) (0.8194, -5.5803) (0.8193, -5.5797) (0.8193, -5.5794) (0.8193, -5.5792) (0.8193, -5.579) (0.8192, -5.579) knots -1 -1 -1 -1 -1 -1 -0.99583333 -0.99166667 -0.9875 -0.98333333 -0.97916667 -0.975 -0.97083333 -0.96666667 -0.9625 -0.95833333 -0.95416667 -0.95 -0.94583333 -0.94166667 -0.9375 -0.93333333 -0.92916667 -0.925 -0.92083333 -0.91666667 -0.9125 -0.90833333 -0.90416667 -0.9 -0.89583333 -0.89166667 -0.8875 -0.88333333 -0.87916667 -0.875 -0.87083333 -0.86666667 -0.8625 -0.85833333 -0.85416667 -0.85 -0.84583333 -0.84166667 -0.8375 -0.83333333 -0.82916667 -0.825 -0.82083333 -0.81666667 -0.8125 -0.80833333 -0.80416667 -0.8 -0.79583333 -0.79166667 -0.7875 -0.78333333 -0.77916667 -0.775 -0.77083333 -0.76666667 -0.7625 -0.75833333 -0.75416667 -0.75 -0.74583333 -0.74166667 -0.7375 -0.73333333 -0.72916667 -0.725 -0.72083333 -0.71666667 -0.7125 -0.70833333 -0.70416667 -0.7 -0.69583333 -0.69166667 -0.6875 -0.68333333 -0.67916667 -0.675 -0.67083333 -0.66666667 -0.6625 -0.65833333 -0.65416667 -0.65 -0.64583333 -0.64166667 -0.6375 -0.63333333 -0.62916667 -0.625 -0.62083333 -0.61666667 -0.6125 -0.60833333 -0.60416667 -0.6 -0.59583333 -0.59166667 -0.5875 -0.58333333 -0.57916667 -0.575 -0.57083333 -0.56666667 -0.5625 -0.55833333 -0.55416667 -0.55 -0.54583333 -0.54166667 -0.5375 -0.53333333 -0.52916667 -0.525 -0.52083333 -0.51666667 -0.5125 -0.50833333 -0.50416667 -0.5 -0.49583333 -0.49166667 -0.4875 -0.48333333 -0.47916667 -0.475 -0.47083333 -0.46666667 -0.4625 -0.45833333 -0.45416667 -0.45 -0.44583333 -0.44166667 -0.4375 -0.43333333 -0.42916667 -0.425 -0.42083333 -0.41666667 -0.4125 -0.40833333 -0.40416667 -0.4 -0.39583333 -0.39166667 -0.3875 -0.38333333 -0.37916667 -0.375 -0.37083333 -0.36666667 -0.3625 -0.35833333 -0.35416667 -0.35 -0.34583333 -0.34166667 -0.3375 -0.33333333 -0.32916667 -0.325 -0.32083333 -0.31666667 -0.3125 -0.30833333 -0.30416667 -0.3 -0.29583333 -0.29166667 -0.2875 -0.28333333 -0.27916667 -0.275 -0.27083333 -0.26666667 -0.2625 -0.25833333 -0.25416667 -0.25 -0.24583333 -0.24166667 -0.2375 -0.23333333 -0.22916667 -0.225 -0.22083333 -0.21666667 -0.2125 -0.20833333 -0.20416667 -0.2 -0.19583333 -0.19166667 -0.1875 -0.18333333 -0.17916667 -0.175 -0.17083333 -0.16666667 -0.1625 -0.15833333 -0.15416667 -0.15 -0.14583333 -0.14166667 -0.1375 -0.13333333 -0.12916667 -0.125 -0.12083333 -0.11666667 -0.1125 -0.10833333 -0.10416667 -0.1 -0.09583333 -0.09166667 -0.0875 -0.08333333 -0.07916667 -0.075 -0.07083333 -0.06666667 -0.0625 -0.05833333 -0.05416667 -0.05 -0.04583333 -0.04166667 -0.0375 -0.03333333 -0.02916667 -0.025 -0.02083333 -0.01666667 -0.0125 -0.00833333 -0.00416667 0 0 0 0 0 0
  line L14 (0.8192, -5.579) -> (0.8192, -5.5783)
  line L15 (0.8192, -5.5783) -> (0.6901, -4.6996)
  arc A8 (0.6901, -4.6996) -> (1.7521, -4.415) centre (0, 0) ccw
  line L16 (1.7521, -4.415) -> (2.0798, -5.2406)
  line L17 (2.0798, -5.2406) -> (2.08, -5.2411)
  spline S8 degree 5 poles (2.08, -5.2411) (2.08, -5.2412) (2.0801, -5.2413) (2.0802, -5.2415) (2.0803, -5.2419) (2.0805, -5.2424) (2.0807, -5.2429) (2.081, -5.2435) (2.0813, -5.2442) (2.0817, -5.245) (2.082, -5.2458) (2.0824, -5.2467) (2.0829, -5.2477) (2.0834, -5.2487) (2.0839, -5.2498) (2.0844, -5.251) (2.085, -5.2522) (2.0856, -5.2535) (2.0863, -5.2549) (2.087, -5.2563) (2.0877, -5.2577) (2.0884, -5.2593) (2.0892, -5.2609) (2.0901, -5.2625) (2.0909, -5.2642) (2.0918, -5.266) (2.0928, -5.2678) (2.0938, -5.2696) (2.0948, -5.2716) (2.0958, -5.2735) (2.0969, -5.2756) (2.0981, -5.2776) (2.0992, -5.2798) (2.1004, -5.2819) (2.1017, -5.2842) (2.1029, -5.2865) (2.1043, -5.2888) (2.1056, -5.2912) (2.107, -5.2936) (2.1084, -5.2961) (2.1099, -5.2986) (2.1114, -5.3012) (2.113, -5.3038) (2.1146, -5.3064) (2.1162, -5.3091) (2.1179, -5.3119) (2.1196, -5.3146) (2.1213, -5.3175) (2.1231, -5.3203) (2.1249, -5.3233) (2.1268, -5.3262) (2.1287, -5.3292) (2.1306, -5.3322) (2.1326, -5.3353) (2.1346, -5.3384) (2.1367, -5.3416) (2.1388, -5.3447) (2.1409, -5.348) (2.1431, -5.3512) (2.1453, -5.3545) (2.1475, -5.3579) (2.1498, -5.3612) (2.1522, -5.3646) (2.1546, -5.3681) (2.157, -5.3715) (2.1594, -5.375) (2.1619, -5.3786) (2.1645, -5.3821) (2.1671, -5.3858) (2.1697, -5.3894) (2.1723, -5.393) (2.175, -5.3967) (2.1778, -5.4005) (2.1806, -5.4042) (2.1834, -5.408) (2.1863, -5.4118) (2.1892, -5.4157) (2.1921, -5.4195) (2.1951, -5.4234) (2.1981, -5.4274) (2.2012, -5.4313) (2.2043, -5.4353) (2.2074, -5.4393) (2.2106, -5.4434) (2.2139, -5.4474) (2.2171, -5.4515) (2.2204, -5.4556) (2.2238, -5.4597) (2.2272, -5.4639) (2.2306, -5.4681) (2.2341, -5.4723) (2.2376, -5.4765) (2.2412, -5.4808) (2.2448, -5.485) (2.2484, -5.4893) (2.2521, -5.4936) (2.2558, -5.498) (2.2596, -5.5023) (2.2634, -5.5067) (2.2673, -5.5111) (2.2711, -5.5155) (2.2751, -5.52) (2.279, -5.5244) (2.283, -5.5289) (2.2871, -5.5334) (2.2912, -5.5379) (2.2953, -5.5424) (2.2995, -5.547) (2.3037, -5.5516) (2.308, -5.5561) (2.3123, -5.5607) (2.3166, -5.5653) (2.321, -5.57) (2.3254, -5.5746) (2.3299, -5.5793) (2.3344, -5.584) (2.3389, -5.5887) (2.3435, -5.5934) (2.3481, -5.5981) (2.3528, -5.6028) (2.3575, -5.6076) (2.3623, -5.6123) (2.3671, -5.6171) (2.3719, -5.6219) (2.3768, -5.6267) (2.3817, -5.6315) (2.3866, -5.6363) (2.3916, -5.6411) (2.3967, -5.646) (2.4017, -5.6508) (2.4068, -5.6557) (2.412, -5.6606) (2.4172, -5.6655) (2.4224, -5.6704) (2.4277, -5.6753) (2.433, -5.6802) (2.4384, -5.6851) (2.4438, -5.69) (2.4492, -5.695) (2.4547, -5.6999) (2.4602, -5.7049) (2.4658, -5.7099) (2.4714, -5.7148) (2.4771, -5.7198) (2.4827, -5.7248) (2.4885, -5.7298) (2.4942, -5.7348) (2.5, -5.7398) (2.5059, -5.7448) (2.5118, -5.7498) (2.5177, -5.7549) (2.5236, -5.7599) (2.5297, -5.7649) (2.5357, -5.77) (2.5418, -5.775) (2.5479, -5.78) (2.5541, -5.7851) (2.5603, -5.7902) (2.5665, -5.7952) (2.5728, -5.8003) (2.5791, -5.8053) (2.5855, -5.8104) (2.5919, -5.8155) (2.5983, -5.8205) (2.6048, -5.8256) (2.6113, -5.8307) (2.6179, -5.8358) (2.6245, -5.8409) (2.6311, -5.8459) (2.6378, -5.851) (2.6445, -5.8561) (2.6513, -5.8612) (2.6581, -5.8663) (2.6649, -5.8714) (2.6718, -5.8764) (2.6787, -5.8815) (2.6857, -5.8866) (2.6927, -5.8917) (2.6997, -5.8968) (2.7068, -5.9019) (2.7139, -5.9069) (2.721, -5.912) (2.7282, -5.9171) (2.7354, -5.9222) (2.7427, -5.9272) (2.75, -5.9323) (2.7573, -5.9374) (2.7647, -5.9424) (2.7721, -5.9475) (2.7796, -5.9526) (2.7871, -5.9576) (2.7946, -5.9627) (2.8022, -5.9677) (2.8098, -5.9728) (2.8174, -5.9778) (2.8251, -5.9828) (2.8328, -5.9879) (2.8406, -5.9929) (2.8484, -5.9979) (2.8562, -6.0029) (2.8641, -6.008) (2.872, -6.013) (2.8799, -6.018) (2.8879, -6.023) (2.8959, -6.0279) (2.904, -6.0329) (2.9121, -6.0379) (2.9202, -6.0429) (2.9284, -6.0478) (2.9366, -6.0528) (2.9448, -6.0577) (2.9531, -6.0627) (2.9614, -6.0676) (2.9698, -6.0726) (2.9782, -6.0775) (2.9866, -6.0824) (2.9951, -6.0873) (3.0036, -6.0922) (3.0121, -6.0971) (3.0207, -6.1019) (3.0293, -6.1068) (3.038, -6.1117) (3.0466, -6.1165) (3.0554, -6.1214) (3.0641, -6.1262) (3.0729, -6.131) (3.0817, -6.1358) (3.0906, -6.1406) (3.0995, -6.1454) (3.1084, -6.1502) (3.1174, -6.155) (3.1264, -6.1598) (3.1354, -6.1645) (3.1445, -6.1692) (3.1536, -6.174) (3.1628, -6.1787) (3.172, -6.1834) (3.1812, -6.1881) (3.1904, -6.1928) (3.1997, -6.1975) (3.209, -6.2021) (3.2165, -6.2058) (3.2221, -6.2086) (3.2259, -6.2105) (3.2278, -6.2114) knots 0 0 0 0 0 0 0.00416667 0.00833333 0.0125 0.01666667 0.02083333 0.025 0.02916667 0.03333333 0.0375 0.04166667 0.04583333 0.05 0.05416667 0.05833333 0.0625 0.06666667 0.07083333 0.075 0.07916667 0.08333333 0.0875 0.09166667 0.09583333 0.1 0.10416667 0.10833333 0.1125 0.11666667 0.12083333 0.125 0.12916667 0.13333333 0.1375 0.14166667 0.14583333 0.15 0.15416667 0.15833333 0.1625 0.16666667 0.17083333 0.175 0.17916667 0.18333333 0.1875 0.19166667 0.19583333 0.2 0.20416667 0.20833333 0.2125 0.21666667 0.22083333 0.225 0.22916667 0.23333333 0.2375 0.24166667 0.24583333 0.25 0.25416667 0.25833333 0.2625 0.26666667 0.27083333 0.275 0.27916667 0.28333333 0.2875 0.29166667 0.29583333 0.3 0.30416667 0.30833333 0.3125 0.31666667 0.32083333 0.325 0.32916667 0.33333333 0.3375 0.34166667 0.34583333 0.35 0.35416667 0.35833333 0.3625 0.36666667 0.37083333 0.375 0.37916667 0.38333333 0.3875 0.39166667 0.39583333 0.4 0.40416667 0.40833333 0.4125 0.41666667 0.42083333 0.425 0.42916667 0.43333333 0.4375 0.44166667 0.44583333 0.45 0.45416667 0.45833333 0.4625 0.46666667 0.47083333 0.475 0.47916667 0.48333333 0.4875 0.49166667 0.49583333 0.5 0.50416667 0.50833333 0.5125 0.51666667 0.52083333 0.525 0.52916667 0.53333333 0.5375 0.54166667 0.54583333 0.55 0.55416667 0.55833333 0.5625 0.56666667 0.57083333 0.575 0.57916667 0.58333333 0.5875 0.59166667 0.59583333 0.6 0.60416667 0.60833333 0.6125 0.61666667 0.62083333 0.625 0.62916667 0.63333333 0.6375 0.64166667 0.64583333 0.65 0.65416667 0.65833333 0.6625 0.66666667 0.67083333 0.675 0.67916667 0.68333333 0.6875 0.69166667 0.69583333 0.7 0.70416667 0.70833333 0.7125 0.71666667 0.72083333 0.725 0.72916667 0.73333333 0.7375 0.74166667 0.74583333 0.75 0.75416667 0.75833333 0.7625 0.76666667 0.77083333 0.775 0.77916667 0.78333333 0.7875 0.79166667 0.79583333 0.8 0.80416667 0.80833333 0.8125 0.81666667 0.82083333 0.825 0.82916667 0.83333333 0.8375 0.84166667 0.84583333 0.85 0.85416667 0.85833333 0.8625 0.86666667 0.87083333 0.875 0.87916667 0.88333333 0.8875 0.89166667 0.89583333 0.9 0.90416667 0.90833333 0.9125 0.91666667 0.92083333 0.925 0.92916667 0.93333333 0.9375 0.94166667 0.94583333 0.95 0.95416667 0.95833333 0.9625 0.96666667 0.97083333 0.975 0.97916667 0.98333333 0.9875 0.99166667 0.99583333 1 1 1 1 1 1
  arc A9 (3.2278, -6.2114) -> (3.7653, -5.901) centre (0, 0) ccw
  spline S9 degree 5 poles (3.7653, -5.901) (3.7655, -5.899) (3.7657, -5.8948) (3.7661, -5.8885) (3.7667, -5.8802) (3.7673, -5.8698) (3.7679, -5.8594) (3.7685, -5.849) (3.769, -5.8387) (3.7695, -5.8284) (3.77, -5.8181) (3.7705, -5.8079) (3.7709, -5.7976) (3.7713, -5.7874) (3.7717, -5.7772) (3.772, -5.7671) (3.7724, -5.757) (3.7727, -5.7468) (3.7729, -5.7368) (3.7732, -5.7267) (3.7734, -5.7167) (3.7736, -5.7067) (3.7738, -5.6967) (3.7739, -5.6868) (3.774, -5.6769) (3.7741, -5.667) (3.7742, -5.6571) (3.7742, -5.6473) (3.7742, -5.6375) (3.7742, -5.6277) (3.7741, -5.6179) (3.7741, -5.6082) (3.774, -5.5985) (3.7739, -5.5888) (3.7737, -5.5792) (3.7736, -5.5696) (3.7734, -5.56) (3.7732, -5.5504) (3.7729, -5.5409) (3.7727, -5.5314) (3.7724, -5.5219) (3.7721, -5.5125) (3.7717, -5.5031) (3.7714, -5.4937) (3.771, -5.4843) (3.7706, -5.475) (3.7702, -5.4657) (3.7697, -5.4565) (3.7692, -5.4472) (3.7687, -5.438) (3.7682, -5.4289) (3.7677, -5.4197) (3.7671, -5.4106) (3.7665, -5.4015) (3.7659, -5.3925) (3.7653, -5.3835) (3.7646, -5.3745) (3.764, -5.3655) (3.7633, -5.3566) (3.7625, -5.3477) (3.7618, -5.3389) (3.761, -5.33) (3.7603, -5.3212) (3.7594, -5.3125) (3.7586, -5.3037) (3.7578, -5.2951) (3.7569, -5.2864) (3.756, -5.2778) (3.7551, -5.2692) (3.7542, -5.2606) (3.7532, -5.2521) (3.7523, -5.2436) (3.7513, -5.2351) (3.7503, -5.2267) (3.7493, -5.2183) (3.7482, -5.2099) (3.7472, -5.2016) (3.7461, -5.1933) (3.745, -5.1851) (3.7439, -5.1768) (3.7427, -5.1687) (3.7416, -5.1605) (3.7404, -5.1524) (3.7392, -5.1443) (3.738, -5.1363) (3.7368, -5.1283) (3.7355, -5.1203) (3.7343, -5.1123) (3.733, -5.1044) (3.7317, -5.0966) (3.7304, -5.0887) (3.7291, -5.081) (3.7277, -5.0732) (3.7264, -5.0655) (3.725, -5.0578) (3.7236, -5.0502) (3.7222, -5.0426) (3.7208, -5.035) (3.7194, -5.0275) (3.7179, -5.02) (3.7165, -5.0125) (3.715, -5.0051) (3.7135, -4.9977) (3.712, -4.9904) (3.7105, -4.9831) (3.7089, -4.9758) (3.7074, -4.9686) (3.7058, -4.9614) (3.7043, -4.9543) (3.7027, -4.9472) (3.7011, -4.9401) (3.6995, -4.9331) (3.6978, -4.9261) (3.6962, -4.9191) (3.6946, -4.9122) (3.6929, -4.9054) (3.6912, -4.8986) (3.6896, -4.8918) (3.6879, -4.885) (3.6862, -4.8783) (3.6845, -4.8717) (3.6827, -4.8651) (3.681, -4.8585) (3.6793, -4.8519) (3.6775, -4.8454) (3.6758, -4.839) (3.674, -4.8326) (3.6722, -4.8262) (3.6705, -4.8199) (3.6687, -4.8136) (3.6669, -4.8074) (3.6651, -4.8012) (3.6632, -4.795) (3.6614, -4.7889) (3.6596, -4.7829) (3.6578, -4.7768) (3.6559, -4.7709) (3.6541, -4.7649) (3.6522, -4.759) (3.6504, -4.7532) (3.6485, -4.7474) (3.6466, -4.7416) (3.6448, -4.7359) (3.6429, -4.7303) (3.641, -4.7246) (3.6391, -4.7191) (3.6373, -4.7135) (3.6354, -4.708) (3.6335, -4.7026) (3.6316, -4.6972) (3.6297, -4.6919) (3.6278, -4.6866) (3.6259, -4.6813) (3.624, -4.6761) (3.6221, -4.6709) (3.6202, -4.6658) (3.6183, -4.6608) (3.6164, -4.6557) (3.6145, -4.6508) (3.6126, -4.6458) (3.6107, -4.641) (3.6088, -4.6361) (3.6069, -4.6314) (3.605, -4.6266) (3.6031, -4.6219) (3.6012, -4.6173) (3.5993, -4.6127) (3.5974, -4.6082) (3.5955, -4.6037) (3.5937, -4.5993) (3.5918, -4.5949) (3.5899, -4.5905) (3.5881, -4.5863) (3.5862, -4.582) (3.5843, -4.5778) (3.5825, -4.5737) (3.5807, -4.5696) (3.5788, -4.5656) (3.577, -4.5616) (3.5752, -4.5577) (3.5734, -4.5538) (3.5716, -4.5499) (3.5698, -4.5462) (3.568, -4.5424) (3.5663, -4.5388) (3.5645, -4.5351) (3.5628, -4.5316) (3.561, -4.5281) (3.5593, -4.5246) (3.5576, -4.5212) (3.5559, -4.5178) (3.5542, -4.5145) (3.5525, -4.5113) (3.5509, -4.5081) (3.5492, -4.5049) (3.5476, -4.5018) (3.546, -4.4988) (3.5444, -4.4958) (3.5428, -4.4929) (3.5413, -4.49) (3.5397, -4.4872) (3.5382, -4.4845) (3.5367, -4.4818) (3.5352, -4.4791) (3.5338, -4.4765) (3.5323, -4.474) (3.5309, -4.4715) (3.5295, -4.4691) (3.5281, -4.4667) (3.5267, -4.4644) (3.5254, -4.4622) (3.5241, -4.46) (3.5228, -4.4579) (3.5215, -4.4558) (3.5203, -4.4538) (3.5191, -4.4518) (3.5179, -4.4499) (3.5168, -4.4481) (3.5156, -4.4463) (3.5145, -4.4446) (3.5135, -4.4429) (3.5124, -4.4413) (3.5114, -4.4398) (3.5104, -4.4383) (3.5095, -4.4369) (3.5086, -4.4355) (3.5077, -4.4342) (3.5069, -4.433) (3.5061, -4.4318) (3.5053, -4.4307) (3.5046, -4.4296) (3.5039, -4.4286) (3.5032, -4.4277) (3.5026, -4.4268) (3.502, -4.426) (3.5015, -4.4253) (3.501, -4.4246) (3.5005, -4.424) (3.5001, -4.4234) (3.4998, -4.423) (3.4994, -4.4225) (3.4992, -4.4222) (3.4991, -4.4221) (3.499, -4.422) (3.499, -4.4219) knots -1 -1 -1 -1 -1 -1 -0.99583333 -0.99166667 -0.9875 -0.98333333 -0.97916667 -0.975 -0.97083333 -0.96666667 -0.9625 -0.95833333 -0.95416667 -0.95 -0.94583333 -0.94166667 -0.9375 -0.93333333 -0.92916667 -0.925 -0.92083333 -0.91666667 -0.9125 -0.90833333 -0.90416667 -0.9 -0.89583333 -0.89166667 -0.8875 -0.88333333 -0.87916667 -0.875 -0.87083333 -0.86666667 -0.8625 -0.85833333 -0.85416667 -0.85 -0.84583333 -0.84166667 -0.8375 -0.83333333 -0.82916667 -0.825 -0.82083333 -0.81666667 -0.8125 -0.80833333 -0.80416667 -0.8 -0.79583333 -0.79166667 -0.7875 -0.78333333 -0.77916667 -0.775 -0.77083333 -0.76666667 -0.7625 -0.75833333 -0.75416667 -0.75 -0.74583333 -0.74166667 -0.7375 -0.73333333 -0.72916667 -0.725 -0.72083333 -0.71666667 -0.7125 -0.70833333 -0.70416667 -0.7 -0.69583333 -0.69166667 -0.6875 -0.68333333 -0.67916667 -0.675 -0.67083333 -0.66666667 -0.6625 -0.65833333 -0.65416667 -0.65 -0.64583333 -0.64166667 -0.6375 -0.63333333 -0.62916667 -0.625 -0.62083333 -0.61666667 -0.6125 -0.60833333 -0.60416667 -0.6 -0.59583333 -0.59166667 -0.5875 -0.58333333 -0.57916667 -0.575 -0.57083333 -0.56666667 -0.5625 -0.55833333 -0.55416667 -0.55 -0.54583333 -0.54166667 -0.5375 -0.53333333 -0.52916667 -0.525 -0.52083333 -0.51666667 -0.5125 -0.50833333 -0.50416667 -0.5 -0.49583333 -0.49166667 -0.4875 -0.48333333 -0.47916667 -0.475 -0.47083333 -0.46666667 -0.4625 -0.45833333 -0.45416667 -0.45 -0.44583333 -0.44166667 -0.4375 -0.43333333 -0.42916667 -0.425 -0.42083333 -0.41666667 -0.4125 -0.40833333 -0.40416667 -0.4 -0.39583333 -0.39166667 -0.3875 -0.38333333 -0.37916667 -0.375 -0.37083333 -0.36666667 -0.3625 -0.35833333 -0.35416667 -0.35 -0.34583333 -0.34166667 -0.3375 -0.33333333 -0.32916667 -0.325 -0.32083333 -0.31666667 -0.3125 -0.30833333 -0.30416667 -0.3 -0.29583333 -0.29166667 -0.2875 -0.28333333 -0.27916667 -0.275 -0.27083333 -0.26666667 -0.2625 -0.25833333 -0.25416667 -0.25 -0.24583333 -0.24166667 -0.2375 -0.23333333 -0.22916667 -0.225 -0.22083333 -0.21666667 -0.2125 -0.20833333 -0.20416667 -0.2 -0.19583333 -0.19166667 -0.1875 -0.18333333 -0.17916667 -0.175 -0.17083333 -0.16666667 -0.1625 -0.15833333 -0.15416667 -0.15 -0.14583333 -0.14166667 -0.1375 -0.13333333 -0.12916667 -0.125 -0.12083333 -0.11666667 -0.1125 -0.10833333 -0.10416667 -0.1 -0.09583333 -0.09166667 -0.0875 -0.08333333 -0.07916667 -0.075 -0.07083333 -0.06666667 -0.0625 -0.05833333 -0.05416667 -0.05 -0.04583333 -0.04166667 -0.0375 -0.03333333 -0.02916667 -0.025 -0.02083333 -0.01666667 -0.0125 -0.00833333 -0.00416667 0 0 0 0 0 0
  line L18 (3.499, -4.4219) -> (3.4986, -4.4214)
  line L19 (3.4986, -4.4214) -> (2.9475, -3.7249)
  arc A10 (2.9475, -3.7249) -> (3.7249, -2.9475) centre (0, 0) ccw
  line L20 (3.7249, -2.9475) -> (4.4214, -3.4986)
  line L21 (4.4214, -3.4986) -> (4.4219, -3.499)